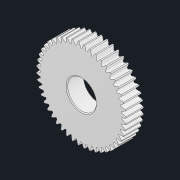
# Autodesk Inventor part: unit-planet_gear
Saved by Autodesk Inventor 2021 (Build 250183000, 183)
## iProperties
Created: 2021-07-12
Part Number: unit-planet_gear
Material: ABS プラスチック
Document SubType Name: Modeling
Designer: yuta0
Density: 1.06 g/cm^3
Appearance: 滑らか - 白
購入先: 印刷
在庫数: 0.0
Author: yuta0
Autodesk Inventor part; units mm, degrees
ref_plane "YZ Plane" through (0, 0, 0) normal (1, 0, 0) x (0, 1, 0)
ref_plane "XZ Plane" through (0, 0, 0) normal (0, 1, 0) x (-1, 0, 0)
ref_plane "XY Plane" through (0, 0, 0) normal (0, 0, 1) x (1, 0, 0)
sketch "スケッチ1" plane through (0, 0, 0) normal (0, 0, 1) x (1, 0, 0)
  spline S0 degree 3 poles (-1.3248, 25.0984) (-1.2679, 24.9945) (-1.154, 24.7867) (-0.997, 24.4677) (-0.8511, 24.1436) (-0.7409, 23.8686) (-0.6602, 23.6457) (-0.6042, 23.4771) (-0.5518, 23.3072) (-0.5154, 23.1637) (-0.4826, 23.0497) (-0.4522, 22.9819) (-0.422, 22.9308) (-0.3957, 22.895) (-0.3669, 22.8611) (-0.3338, 22.8314) (-0.2985, 22.8042) (-0.2599, 22.782) (-0.2196, 22.7631) (-0.1767, 22.7514) (-0.1334, 22.741) (-0.074, 22.7383) (0, 22.7398) (0.074, 22.7383) (0.1334, 22.741) (0.1767, 22.7514) (0.2196, 22.7631) (0.2599, 22.782) (0.2985, 22.8042) (0.3338, 22.8314) (0.3669, 22.8611) (0.3957, 22.895) (0.422, 22.9308) (0.4522, 22.9819) (0.4826, 23.0497) (0.5154, 23.1637) (0.5518, 23.3072) (0.6042, 23.4771) (0.6602, 23.6457) (0.7409, 23.8686) (0.8511, 24.1436) (0.997, 24.4677) (1.154, 24.7867) (1.2679, 24.9945) (1.3248, 25.0984) knots 0 0 0 0 0.035541 0.071082 0.106623 0.142163 0.159934 0.177705 0.195476 0.213247 0.222131 0.231011 0.235454 0.239896 0.244338 0.24878 0.25322 0.257663 0.262105 0.266544 0.270985 0.275428 0.284313 0.293199 0.297641 0.302082 0.306522 0.310964 0.315406 0.319846 0.324289 0.328731 0.333172 0.337616 0.346496 0.355379 0.37315 0.390921 0.408692 0.426463 0.462003 0.497544 0.533085 0.568626 0.568626 0.568626 0.568626
  circle A0 centre (0, 0) radius 22.7392 construction
  circle A1 centre (0, 0) radius 22.5526 construction
  circle A2 centre (0, 0) radius 24 construction
  circle A3 centre (0, 0) radius 25.1333
  point P0 (-1.1563, 24.7855)
  point P1 (-0.9988, 24.4669)
  point P2 (-0.8533, 24.1426)
  point P3 (-0.7213, 23.8126)
  point P4 (-0.661, 23.6455)
  point P5 (-0.6048, 23.4769)
  point P6 (-0.5533, 23.3068)
  point P7 (-0.5069, 23.1352)
  point P8 (-0.4806, 23.0504)
  point P9 (-0.4442, 22.9694)
  point P10 (-0.4214, 22.9312)
  point P11 (-0.3953, 22.8953)
  point P12 (-0.3662, 22.8618)
  point P13 (-0.3334, 22.8318)
  point P14 (-0.298, 22.805)
  point P15 (-0.2596, 22.7826)
  point P16 (-0.2192, 22.7643)
  point P17 (-0.1766, 22.7516)
  point P18 (-0.1332, 22.7424)
  point P19 (-0.0889, 22.7393)
  point P20 (0, 22.7392)
  point P21 (0.0889, 22.7393)
  point P22 (0.1332, 22.7424)
  point P23 (0.1766, 22.7516)
  point P24 (0.2192, 22.7643)
  point P25 (0.2596, 22.7826)
  point P26 (0.298, 22.805)
  point P27 (0.3334, 22.8318)
  point P28 (0.3662, 22.8618)
  point P29 (0.3953, 22.8953)
  point P30 (0.4214, 22.9312)
  point P31 (0.4442, 22.9694)
  point P32 (0.4806, 23.0504)
  point P33 (0.5069, 23.1352)
  point P34 (0.5533, 23.3068)
  point P35 (0.6048, 23.4769)
  point P36 (0.661, 23.6455)
  point P37 (0.7213, 23.8126)
  point P38 (0.8533, 24.1426)
  point P39 (0.9988, 24.4669)
  point P40 (1.1563, 24.7855)
  constraints: 4 centre point, 2 point on circle, 91 other
extrude "押し出し1" add sketch "スケッチ1" along normal mid plane 9.8
extrude "押し出し3" cut sketch "スケッチ1" along normal through all both and the other way through all contours A3 S0 picked at (-0.0654, 24.1816)
sketch "スケッチ3" plane through (0, 0, 0) normal (0, 1, 0) x (-1, 0, 0)
  line L0 (25.1333, 4.4) -> (24.6333, 4.9)
  line L1 (25.1333, 0) -> (-25.1333, 0) projected
  line L2 (8.55, 4.9) -> (-8.55, 4.9) projected
  line L3 (25.1333, 4.4) -> (25.1333, 4.9)
  line L4 (25.1333, 4.9) -> (24.6333, 4.9)
  line L5 (0, -6.8643) -> (0, 6.8643) projected
  point P0 (0, 0)
  dimension "d13" = 45
  dimension "d14" = 0.5
  constraints: 6 end point, 1 horizontal alignment, 1 perpendicular, 1 vertical, 1 vertical alignment
  measures "d13" angle of L0 L1
  measures "d14" horizontal distance of L0.start L0.end
pattern_circular "円形状パターン1" count 48 over 360 about axis through (0, 0, -10) along (0, 0, 1) of "押し出し3"
sketch "スケッチ2" plane through (0, 0, 4.9) normal (0, 0, 1) x (1, 0, 0)
  circle A0 centre (0, 0) radius 8.05
  dimension "d2" = 16.1
  constraints: 1 centre point, 1 coincident
  measures "d2" diameter of A0
extrude "押し出し2" cut sketch "スケッチ2" against normal through all
chamfer "面取り1" distance 0.5 angle 45 2 edges at (-8.05, 0, 4.9) (-8.05, 0, -4.9)
